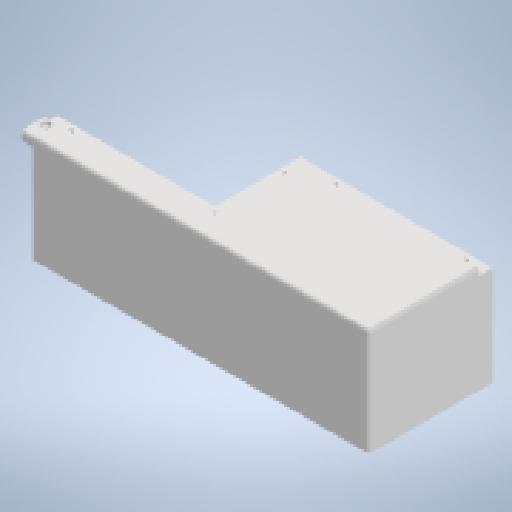
# Autodesk Inventor part: オンゲキボタン_top1
Saved by Autodesk Inventor 2025.2 (Build 292293000, 293)
## iProperties
Created: 2025-05-09
Part Number: オンゲキボタン_top1
Material: 一般
Document SubType Name: Modeling
Designer: mahhy
Density: 1 g/cm^3
Appearance: 既定
Author: mahhy
## iProperties of the stored document オンゲキボタン_top1_3D プリント.ipt
Created: 2025-05-14
Part Number: オンゲキボタン_top1_3D プリント
Material: 一般
Document SubType Name: Modeling
Designer: mahhy
Density: 1 g/cm^3
Appearance: 既定
Author: mahhy
Autodesk Inventor part; units mm, degrees
ref_plane "YZ Plane" through (0, 0, 0) normal (1, 0, 0) x (0, 1, 0)
ref_plane "XZ Plane" through (0, 0, 0) normal (0, 1, 0) x (-1, 0, 0)
ref_plane "XY Plane" through (0, 0, 0) normal (0, 0, 1) x (1, 0, 0)
sketch "スケッチ1" plane through (0, 0, 0) normal (0, 1, 0) x (-1, 0, 0)
  line L0 (0, 0) -> (204, 0)
  line L1 (204, 0) -> (204, -72)
  line L2 (204, -72) -> (0, -72)
  line L3 (0, -72) -> (0, 0)
  dimension "d0" = 204
  dimension "d1" = 72
  constraints: 8 end point, 2 parallel, 1 horizontal, 1 perpendicular
  measures "d0" distance of L1.end L2.end
  measures "d1" distance of L0.end L1.end
extrude "押し出し1" add sketch "スケッチ1" along normal blind 7
sketch "スケッチ2" plane through (0, 7, 0) normal (0, 1, 0) x (1, 0, 0)
  line L0 (-204, 22) -> (-112, 22)
  line L1 (-112, 22) -> (-112, 72)
  line L2 (-112, 72) -> (-204, 72)
  line L3 (-204, 72) -> (-204, 22)
  line L4 (-204, 72) -> (-204, 0) projected
  line L5 (0, 72) -> (-204, 72) projected
  line L6 (-204, 0) -> (0, 0) projected
  dimension "d5" = 92
  dimension "d76" = 50
  constraints: 8 end point, 2 collinear, 2 parallel, 1 horizontal, 1 perpendicular
  measures "d5" distance of L1.end L2.end
  measures "d76" distance of L2.end L0.start
extrude "押し出し2" cut sketch "スケッチ2" against normal through all
sketch "スケッチ3" plane through (0, 7, 0) normal (0, 1, 0) x (1, 0, 0)
  line L0 (-204, 22) -> (-204, 0) projected
  line L1 (-204, 22) -> (-112, 22)
  line L2 (-112, 22) -> (-112, 14)
  line L3 (-112, 14) -> (-204, 14)
  line L4 (-204, 14) -> (-204, 22)
  line L5 (-112, 72) -> (-112, 22) projected
  line L6 (-112, 72) -> (-104, 72)
  line L7 (-104, 72) -> (-104, 14)
  line L8 (-104, 14) -> (-112, 14)
  line L9 (-112, 14) -> (-112, 72)
  line L10 (0, 72) -> (-112, 72) projected
  line L11 (0, 0) -> (0, 72) projected
  line L12 (-112, 72) -> (0, 72)
  line L13 (0, 72) -> (0, 64)
  line L14 (0, 64) -> (-112, 64)
  line L15 (-112, 64) -> (-112, 72)
  point P0 (-204, 14)
  point P1 (-104, 64)
  dimension "d8" = 8
  dimension "d9" = 8
  dimension "d19" = 8
  constraints: 24 end point, 6 parallel, 3 horizontal, 3 perpendicular, 2 point on line
  measures "d8" distance of L1.end L2.end
  measures "d9" distance of L7.end L8.end
  measures "d19" distance of L12.end L13.end
extrude "押し出し3" cut sketch "スケッチ3" against normal blind 4
sketch "スケッチ4" plane through (0, 3, 0) normal (0, 1, 0) x (1, 0, 0)
  circle A0 centre (-192, 18) radius 1.5
  circle A1 centre (-108, 18) radius 1.5
  circle A2 centre (-108, 59) radius 1.5
  line L0 (-112, 72) -> (0, 72) projected
  line L1 (-204, 14) -> (-204, 22) projected
  line L2 (-112, 22) -> (-112, 72) projected
  circle A3 centre (-88, 68) radius 1.5
  circle A4 centre (-12, 68) radius 1.5
  line L3 (0, 72) -> (0, 64) projected
  point P0 (0, 0)
  point P1 (-204, 18)
  point P2 (-204, 18)
  dimension "d12" = 3
  dimension "d13" = 3
  dimension "d14" = 3
  dimension "d16" = 12
  dimension "d20" = 4
  dimension "d21" = 3
  dimension "d22" = 3
  dimension "d23" = 4
  dimension "d24" = 24
  dimension "d25" = 12
  dimension "d32" = 41
  dimension "d34" = 76
  constraints: 5 centre point, 3 horizontal alignment, 2 midpoint, 1 vertical alignment
  measures "d12" diameter of A0
  measures "d13" diameter of A1
  measures "d14" diameter of A2
  measures "d16" distance of point (-204, 18) A0.centre
  measures "d20" distance from line of L2 A2.centre
  measures "d21" diameter of A3
  measures "d22" diameter of A4
  measures "d23" distance from line of L0 A3.centre
  measures "d24" distance from line of L2 A3.centre
  measures "d25" distance from line of L3 A4.centre
  measures "d32" distance of A1.centre A2.centre
  measures "d34" distance of A4.centre A3.centre
extrude "押し出し4" cut sketch "スケッチ4" against normal through all
sketch "スケッチ5" plane through (0, 0, 0) normal (0, -1, 0) x (1, 0, 0)
  line L0 (-204, 0) -> (0, 0) projected
  line L1 (-204, -22) -> (-112, -22) projected
  line L2 (-204, 0) -> (-196, 0)
  line L3 (-196, 0) -> (-196, -22)
  line L4 (-196, -22) -> (-204, -22)
  line L5 (-204, -22) -> (-204, 0)
  dimension "d26" = 8
  constraints: 8 end point, 2 parallel, 1 horizontal, 1 perpendicular, 1 point on line
  measures "d26" distance of L3.end L4.end
extrude "押し出し5" cut sketch "スケッチ5" against normal blind 2
sketch "スケッチ6" plane through (0, 0, 0) normal (0, -1, 0) x (1, 0, 0)
  line L0 (-196, 0) -> (-196, -22) projected
  line L1 (0, 0) -> (-196, 0)
  line L2 (-196, 0) -> (-196, -5)
  line L3 (-196, -5) -> (0, -5)
  line L4 (0, -5) -> (0, 0)
  line L5 (-196, 0) -> (0, 0) projected
  line L6 (-112, -72) -> (0, -72) projected
  line L7 (0, 0) -> (-5, 0)
  line L8 (-5, 0) -> (-5, -72)
  line L9 (-5, -72) -> (0, -72)
  line L10 (0, -72) -> (0, 0)
  point P0 (0, -72)
  point P1 (-5, -5)
  dimension "d29" = 5
  dimension "d33" = 5
  constraints: 16 end point, 4 parallel, 2 horizontal, 2 perpendicular, 2 point on line
  measures "d29" distance of L2.end L1.end
  measures "d33" distance of L9.end L8.end
extrude "押し出し6" add sketch "スケッチ6" along normal blind 55
fillet "フィレット1" radius 2 4 edges at (-102, 7, 0) (0, 7, -32) (0, -24, 0) (-204, 7, -7)
sketch "スケッチ7" plane through (-5, 0, -5) normal (0, 0, -1) x (-1, 0, 0)
  line L0 (191, 2) -> (191, -55) projected
  line L1 (0, 0) -> (191, 0) projected
  line L2 (191, -55) -> (181, -55)
  line L3 (181, -55) -> (181, 0)
  line L4 (181, 0) -> (191, 0)
  line L5 (191, 0) -> (191, -55)
  point P0 (-5, 0)
  dimension "d36" = 10
  constraints: 8 end point, 2 parallel, 1 horizontal, 1 perpendicular, 1 point on line
  measures "d36" distance of L3.end L4.end
extrude "押し出し7" add sketch "スケッチ7" along normal blind 3
sketch "スケッチ8" plane through (-196, 2, -22) normal (-1, 0, 0) x (0, 0, 1)
  circle A0 centre (18, -41) radius 1.5
  circle A1 centre (18, -8) radius 1.5
  line L0 (22, -57) -> (14, -57) projected
  line L1 (0, 0) -> (22, 0) projected
  point P0 (22, -2)
  point P1 (18, -57)
  point P2 (18, -57)
  dimension "d39" = 3
  dimension "d40" = 3
  dimension "d41" = 16
  dimension "d62" = 8
  constraints: 2 centre point, 2 midpoint, 2 vertical alignment
  measures "d39" diameter of A0
  measures "d40" diameter of A1
  measures "d41" vertical distance of L0.start A0.centre
  measures "d62" distance from line of L1 A1.centre
extrude "押し出し8" cut sketch "スケッチ8" against normal blind 8
sketch "スケッチ9" plane through (0, -55, 0) normal (0, -1, 0) x (1, 0, 0)
  line L0 (-5, -5) -> (-5, -72) projected
  circle A0 centre (-5, -5) radius 3
  circle A1 centre (-5, -64) radius 3
  line L1 (-186, -5) -> (-5, -5) projected
  circle A2 centre (-101, -5) radius 3
  circle A3 centre (-191, -5) radius 3
  line L2 (-5, -72) -> (0, -72) projected
  point P0 (0, 0)
  dimension "d45" = 6
  dimension "d46" = 6
  dimension "d47" = 6
  dimension "d48" = 96
  dimension "d49" = 6
  dimension "d50" = 90
  dimension "d78" = 8
  constraints: 4 centre point, 3 point on line
  measures "d45" diameter of A0
  measures "d46" diameter of A1
  measures "d47" diameter of A2
  measures "d48" distance of A2.centre L0.start
  measures "d49" diameter of A3
  measures "d50" distance of A3.centre A2.centre
  measures "d78" distance from line of L2 A1.centre
extrude "押し出し9" add sketch "スケッチ9" against normal blind 15 contours L1 A0 L0 | L0 A0 L1 | A1 L0 | L0 A1 | A2 L1 | L1 A2
sketch "スケッチ10" plane through (0, -55, 0) normal (0, -1, 0) x (1, 0, 0)
  line L0 (-5, -5) -> (-186, -5) projected
  circle A0 centre (-5, -5) radius 1.5
  line L1 (-98, -5) -> (-104, -5) projected
  circle A1 centre (-101, -5) radius 1.5
  arc A2 (-5, -61) -> (-5, -67) centre (-5, -64) ccw projected
  circle A3 centre (-5, -64) radius 1.5
  circle A4 centre (-189, -5) radius 1.5
  line L2 (-186, -8) -> (-196, -8) projected
  line L3 (-186, -5) -> (-186, -8) projected
  point P0 (0, 0)
  dimension "d54" = 3
  dimension "d55" = 3
  dimension "d56" = 3
  dimension "d57" = 3
  dimension "d58" = 3
  dimension "d59" = 3
  constraints: 4 centre point, 1 coincident, 1 midpoint
  measures "d54" diameter of A0
  measures "d55" diameter of A1
  measures "d56" diameter of A3
  measures "d57" diameter of A4
  measures "d58" distance from line of L2 A4.centre
  measures "d59" distance from line of L3 A4.centre
extrude "押し出し10" cut sketch "スケッチ10" against normal blind 12
sketch "スケッチ11" plane through (0, 7, 0) normal (0, 1, 0) x (1, 0, 0)
  circle A0 centre (-198.5, 10) radius 2.8
  line L0 (-204, 14) -> (-204, 0) projected
  line L1 (-204, 0) -> (-2, 0) projected
  line L2 (-104, 14) -> (-202, 14) projected
  line L3 (-202, 2) -> (-202, 14) projected
  point P0 (0, 0)
  dimension "d63" = 5.6
  dimension "d65" = 5.5
  dimension "d77" = 4
  dimension "d79" = 10
  constraints: 1 centre point
  measures "d63" diameter of A0
  measures "d65" distance from line of L0 A0.centre
  measures "d77" distance from line of L2 A0.centre
  measures "d79" distance from line of L1 A0.centre
extrude "押し出し11" cut sketch "スケッチ11" against normal blind 2.5
sketch "スケッチ12" plane through (-198.5, 4.5, -10) normal (0, 1, 0) x (1, 0, 0)
  line L0 (2.5, -10) -> (2.5, 12) projected
  circle A0 centre (0, 0) radius 1.5
  circle A1 centre (0, 0) radius 2.8 projected
  point P0 (198.5, -10)
  dimension "d71" = 3
  constraints: 2 coincident, 1 centre point
  measures "d71" diameter of A0
extrude "押し出し12" cut sketch "スケッチ12" against normal through all contours A0
fillet "フィレット2" radius 2 2 edges at (-203.4142, 6.4142, -0.5858) (-204, 3.5, 0)
